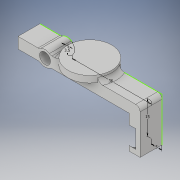
# Autodesk Inventor part: Rocker1
Saved by Autodesk Inventor 2019 (Build 230136000, 136)
## iProperties
Created: 2019-01-13
Part Number: Rocker1
Material: Generic
Document SubType Name: Modeling
Designer: Kepler
Density: 1 g/cm^3
Appearance: Default
Author: Kepler
Autodesk Inventor part; units mm, degrees
note: some values were not read from the file. Chosen so that the rebuilt part matches the saved one: edges of "Fillet2".
ref_plane "YZ Plane" through (0, 0, 0) normal (1, 0, 0) x (0, 1, 0)
ref_plane "XZ Plane" through (0, 0, 0) normal (0, 1, 0) x (-1, 0, 0)
ref_plane "XY Plane" through (0, 0, 0) normal (0, 0, 1) x (1, 0, 0)
sketch "Sketch1" plane through (0, 0, 0) normal (0, 0, 1) x (1, 0, 0)
  line L0 (0, 0) -> (9.8884, 0)
  line L1 (9.8884, 5) -> (0, 5)
  line L2 (0, 5) -> (0, 0)
  circle A0 centre (12.3379, 2.5) radius 2.5
  line L3 (14.7874, 5) -> (19.5284, 5)
  arc A1 (14.7874, 5) -> (9.8884, 5) centre (12.3379, 2.5) ccw
  arc A2 (9.8884, 0) -> (14.7874, 0) centre (12.3379, 2.5) ccw
  line L4 (19.5284, 5) -> (55.7874, 5)
  line L5 (14.7874, 0) -> (50.7874, 0)
  line L6 (50.7874, 0) -> (50.7874, -15)
  line L7 (50.7874, -15) -> (55.7874, -15)
  line L8 (55.7874, -15) -> (55.7874, 5)
  dimension "d6" = 5
  dimension "d7" = 3.5
  dimension "d8" = 36
  dimension "d9" = 15
  dimension "d10" = 5
  constraints: 18 end point, 4 perpendicular, 4 point on circle, 3 centre point, 3 horizontal, 1 coincident, 1 point on line
  measures "d6" diameter of A0
  measures "d7" radius of A1
  measures "d8" distance of L5.start L5.end
  measures "d9" distance of L5.end L6.end
  measures "d10" distance of L6.end L7.end
extrude "Extrusion1" add sketch "Sketch1" along normal blind 10
sketch "Sketch2" plane through (14.7874, 5, 0) normal (0, 1, 0) x (1, 0, 0)
  circle A0 centre (13.0191, -5) radius 10
  point P0 (-14.7874, 0)
  dimension "d16" = 20
  constraints: 1 centre point
  measures "d16" diameter of A0
extrude "Extrusion2" add sketch "Sketch2" along normal blind 3
fillet "Fillet1" radius 2 1 edges at (17.8065, 5, 5)
fillet "Fillet2" radius 2 1 edges at (37.4658, 5, 2.4118)
fillet "Fillet3" radius 2 1 edges at (55.7874, 5, 5)
sketch "Sketch3" plane through (50.7874, -15, 0) normal (-1, 0, 0) x (0, 0, 1)
  circle A0 centre (4.8232, 6.283) radius 6.592
  line L0 (0, 0) -> (10, 0) projected
  point P0 (0, 15)
  constraints: 1 centre point
extrude "Extrusion3" cut sketch "Sketch3" against normal blind 3
fillet "Fillet4" radius 2 1 edges at (14.7874, 5, 5)
fillet "Fillet5" radius 2 1 edges at (9.8884, 5, 5)
fillet "Fillet6" radius 2 1 edges at (14.7874, 0, 5)
fillet "Fillet7" radius 2 1 edges at (9.8884, 0, 5)
sketch "Sketch4" plane through (0, 0, 0) normal (-1, 0, 0) x (0, 0, 1)
  point P0 (0, 0)
  point P1 (5.1471, 2.6969)
hole "Hole1" at (0, 2.6969, 5.1471) direction (1, 0, 0) diameter 2 depth 2 tip angle 118
body "Solid1"
